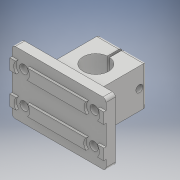
# Autodesk Inventor part: CarroZ - FusoZ
Saved by Autodesk Inventor 2017 (Build 210142000, 142)
## iProperties
Created: 2020-08-03
Part Number: CarroZ - FusoZ
Material: Generic
Document SubType Name: Modeling
Designer: ale
Density: 1 g/cm^3
Appearance: Default
Author: ale
Autodesk Inventor part; units mm, degrees
ref_plane "YZ Plane" through (0, 0, 0) normal (1, 0, 0) x (0, 1, 0)
ref_plane "XZ Plane" through (0, 0, 0) normal (0, 1, 0) x (-1, 0, 0)
ref_plane "XY Plane" through (0, 0, 0) normal (0, 0, 1) x (1, 0, 0)
sketch "Sketch1" plane through (0, 0, 0) normal (0, 0, 1) x (1, 0, 0)
  arc A0 (-0.7641, 8.1141) -> (0.7641, 8.1141) centre (0, 0) ccw
  line L0 (15, 17.5) -> (15, -17.5)
  line L1 (15, -17.5) -> (-15, -17.5)
  line L2 (-15, -17.5) -> (-15, 17.5)
  line L3 (-15, 17.5) -> (15, -17.5) construction
  line L4 (15, 17.5) -> (-15, -17.5) construction
  line L5 (-0.7641, 8.1141) -> (-0.7641, 17.5)
  line L6 (0.7641, 8.1141) -> (0.7641, 17.5)
  line L7 (-15, 17.5) -> (-0.7641, 17.5)
  line L8 (0.7641, 17.5) -> (15, 17.5)
  dimension "d0" = 16.3
  dimension "d1" = 30
  dimension "d2" = 35
  dimension "d26" = 35
  constraints: 18 end point, 3 parallel, 2 horizontal, 2 midpoint, 2 perpendicular, 2 point on circle, 1 centre point, 1 coincident
  measures "d0" diameter of A0
  measures "d1" distance of L0.end L1.end
  measures "d2" distance of L0.start L0.end
  measures "d26" distance between parallel lines of L7 L1
extrude "Extrusion1" add sketch "Sketch1" along normal blind 25
sketch "Sketch2" plane through (-15, -17.5, 0) normal (0, -1, 0) x (1, 0, 0)
  line L0 (15, 0) -> (15, 25)
  line L1 (6.85, 25) -> (23.15, 25) projected
  line L2 (45, 32.5) -> (-15, 32.5)
  line L3 (-15, 32.5) -> (-15, -7.5)
  line L4 (-15, -7.5) -> (45, -7.5)
  line L5 (45, -7.5) -> (45, 32.5)
  line L6 (45, 32.5) -> (-15, -7.5) construction
  line L7 (-15, 32.5) -> (45, -7.5) construction
  point P0 (15.7641, 25)
  point P1 (14.2359, 25)
  point P2 (15, 12.5)
  dimension "d7" = 60
  dimension "d8" = 40
  constraints: 14 end point, 4 midpoint, 2 parallel, 1 horizontal, 1 perpendicular
  measures "d7" distance of L4.end L3.end
  measures "d8" distance of L3.end L2.end
extrude "Extrusion2" add sketch "Sketch2" along normal blind 6
sketch "Sketch4" plane through (-15, -23.5, 0) normal (0, -1, 0) x (1, 0, 0)
  line L0 (-15, 32.5) -> (-15, -7.5) projected
  line L1 (45, -7.5) -> (45, 32.5) projected
  line L2 (-15, -1) -> (45, -1)
  line L3 (-15, 6) -> (45, 6)
  line L4 (-15, 19) -> (45, 19)
  line L5 (-15, 26) -> (45, 26)
  line L6 (-15, -1) -> (-15, 6)
  line L7 (-15, 19) -> (-15, 26)
  line L8 (45, 26) -> (45, 19)
  line L9 (45, 6) -> (45, -1)
  point P0 (15, 0)
  constraints: 16 end point, 4 collinear
extrude "Extrusion3" add sketch "Sketch4" along normal blind 1.5 contours L5 L1 L4 L0 | L3 L1 L2 L0
sketch "Sketch5" plane through (-15, -25, 0) normal (0, -1, 0) x (1, 0, 0)
  line L0 (-14.5701, -1.0846) -> (0, 6)
  line L1 (45, 6) -> (-15, 6) projected
  line L2 (0, 0) -> (0, 25) projected
  line L3 (-15, 19) -> (45, 19) projected
  line L4 (-15, 19) -> (0, 26.2937)
  line L5 (15, 0) -> (15, 25)
  line L6 (6.85, 25) -> (23.15, 25) projected
  line L7 (44.5701, -1.0846) -> (30, 6)
  line L8 (45, 19) -> (30, 26.2937)
  point P0 (-7.285, 2.4577)
  point P1 (-7.5, 22.6468)
  point P2 (15.7641, 25)
  point P3 (14.2359, 25)
  point P4 (37.285, 2.4577)
  point P5 (37.5, 22.6468)
  constraints: 10 end point, 5 symmetric about line, 3 midpoint, 2 point on line, 1 parallel
hole "Hole1" at (-22.285, -25, 2.4577) at (-22.5, -25, 22.6468) at (22.285, -25, 2.4577) at (22.5, -25, 22.6468) direction (0, 1, 0) diameter 5.5 end through all counterbore diameter 10 counterbore depth 1.5
sketch "Sketch6" plane through (-15, 17.5, 0) normal (-1, 0, 0) x (0, 0, 1)
  line L0 (25, 0) -> (25, -35) projected
  line L1 (0, -9.3859) -> (25, -9.3859) projected
  line L2 (25, 0) -> (0, -9.3859)
  point P0 (0, -17.5)
  point P1 (12.5, -4.6929)
  constraints: 2 end point, 1 midpoint
hole "Hole2" at (-15, 12.8071, 12.5) direction (1, 0, 0) diameter 4.5 end through all
fillet "Fillet1" radius 2 10 edges at (30, -20.5, -7.5) (-30, -20.5, -7.5) (-15, 17.5, 12.5) (-7.882, 17.5, 0) (7.882, 17.5, 0) (7.882, 17.5, 25) (-7.882, 17.5, 25) (15, 17.5, 12.5) (30, -20.5, 32.5) (-30, -20.5, 32.5)
body "Solid1"
